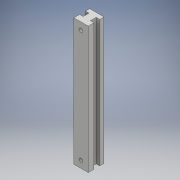
# Autodesk Inventor part: Screen Docking rail
Saved by Autodesk Inventor 2018 (Build 220112000, 112)
## iProperties
Created: 2018-05-10
Part Number: Screen Docking rail
Material: Generic
Document SubType Name: Modeling
Designer: Jasper
Density: 1 g/cm^3
Appearance: Default
Author: Jasper
Autodesk Inventor part; units mm, degrees
ref_plane "YZ Plane" through (0, 0, 0) normal (1, 0, 0) x (0, 1, 0)
ref_plane "XZ Plane" through (0, 0, 0) normal (0, 1, 0) x (-1, 0, 0)
ref_plane "XY Plane" through (0, 0, 0) normal (0, 0, 1) x (1, 0, 0)
sketch "Sketch1" plane through (0, 0, 0) normal (0, 1, 0) x (-1, 0, 0)
  line L0 (-5, 44.25) -> (5, 44.25)
  line L1 (5, 44.25) -> (5, -44.25)
  line L2 (5, -44.25) -> (-5, -44.25)
  line L3 (-5, -44.25) -> (-5, 44.25)
  line L4 (-5, 44.25) -> (5, -44.25) construction
  line L5 (5, 44.25) -> (-5, -44.25) construction
  point P0 (0, 0)
  dimension "d0" = 88.5
  dimension "d1" = 10
  constraints: 12 end point, 2 midpoint, 2 parallel, 1 horizontal, 1 perpendicular
  measures "d0" distance of L0.end L1.end
  measures "d1" distance of L1.end L2.end
extrude "Extrusion1" add sketch "Sketch1" along normal blind 11
sketch "Sketch2" plane through (-5, 0, 44.25) normal (0, 0, 1) x (1, 0, 0)
  line L0 (10, 0) -> (0, 0) projected
  line L1 (5, 0) -> (0, 0)
  line L2 (0, 0) -> (0, 4)
  line L3 (0, 4) -> (2.5, 4)
  line L4 (2.5, 4) -> (2.5, 8)
  line L5 (2.5, 8) -> (0, 8)
  line L6 (0, 8) -> (0, 11)
  line L7 (0, 11) -> (5, 11)
  line L8 (0, 11) -> (10, 11) projected
  line L9 (5, 11) -> (5, 0) construction
  line L10 (0, 0) -> (10, 0)
  line L11 (10, 0) -> (10, 4)
  line L12 (10, 4) -> (7.5, 4)
  line L13 (7.5, 4) -> (7.5, 8)
  line L14 (7.5, 8) -> (10, 8)
  line L15 (10, 8) -> (10, 11)
  line L16 (10, 11) -> (5, 11)
  dimension "d4" = 3
  dimension "d5" = 4
  dimension "d6" = 2.5
  constraints: 30 end point, 7 symmetric about line, 4 perpendicular, 4 point on line, 2 horizontal, 2 midpoint, 1 vertical
  measures "d4" distance of L6.end L5.end
  measures "d5" distance of L0.end L2.end
  measures "d6" distance of L2.end L3.end
extrude "Extrusion2" cut sketch "Sketch2" against normal through all keep common part
sketch "Sketch3" plane through (0, 0, 0) normal (0, -1, 0) x (1, 0, 0)
  line L0 (0, 0) -> (0, 39.25) construction
  circle A0 centre (0, 39.25) radius 1.25
  line L1 (5, -44.25) -> (5, 44.25) construction
  line L2 (5, 0) -> (-5, 0) construction
  line L3 (-5, 44.25) -> (-5, -44.25) construction
  circle A1 centre (0, -39.25) radius 1.25
  dimension "d9" = 2.5
  dimension "d10" = 39.25
  constraints: 4 end point, 2 centre point, 2 midpoint, 1 coincident, 1 symmetric about line, 1 vertical, 1 other
  measures "d9" diameter of A0
  measures "d10" distance of L0.start L0.end
extrude "Extrusion3" cut sketch "Sketch3" against normal blind 4
sketch "Sketch4" plane through (0, 11, 0) normal (0, 1, 0) x (1, 0, 0)
  line L0 (-2, 11) -> (2, 11)
  line L1 (2, 11) -> (2, -9)
  line L2 (2, -9) -> (-2, -9)
  line L3 (-2, -9) -> (-2, 11)
  line L4 (-2, 11) -> (2, -9) construction
  line L5 (2, 11) -> (-2, -9) construction
  line L6 (0, 1) -> (0, 0) construction
  dimension "d13" = 4
  dimension "d14" = 20
  dimension "d15" = 1
  constraints: 14 end point, 2 midpoint, 2 parallel, 1 horizontal, 1 perpendicular, 1 vertical
  measures "d13" distance of L0.start L0.end
  measures "d14" distance of L2.end L0.start
  measures "d15" distance of L6.start L6.end
extrude "Extrusion4" cut sketch "Sketch4" against normal blind 4.7
sketch "Sketch5" plane through (0, 11, 0) normal (0, 1, 0) x (1, 0, 0)
  line L0 (-2, -9) -> (-2, 11) projected
  line L1 (-2, 11) -> (2, 11) projected
  line L2 (2, 11) -> (2, -9) projected
  line L3 (-1.5, -9) -> (-1.5, 10.5)
  line L4 (-1.5, 10.5) -> (1.5, 10.5)
  line L5 (1.5, 10.5) -> (1.5, -9)
  line L6 (-1.5, -9) -> (1.5, -9)
  line L7 (2, -9) -> (-2, -9) projected
  point P0 (0, 0)
  dimension "d18" = 0.5
  constraints: 8 end point, 1 collinear, 1 horizontal, 2 other
  measures "d18" distance between parallel lines of L0 L3
extrude "Extrusion5" add sketch "Sketch5" against normal blind 0.6 contours L3 L4 L5 L6
fillet "Fillet1" radius 4 1 edges at (0, 10.4, 9)
sketch "Sketch7" plane through (0, 11, 0) normal (0, 1, 0) x (1, 0, 0)
  line L0 (1.5, 10.5) -> (-1.5, 10.5) construction
  line L1 (-1.5, 10.5) -> (1.5, 10.5) construction
  line L2 (1.5, 10.5) -> (1.5, 7.5) construction
  line L3 (1.5, 7.5) -> (-1.5, 7.5) construction
  line L4 (-1.5, 7.5) -> (-1.5, 10.5) construction
  line L5 (1.5, -9) -> (1.5, 10.5) projected
  line L6 (-1.5, 10.5) -> (1.5, 7.5) construction
  circle A0 centre (0, 9) radius 1.5
  line L7 (0, 9) -> (1.5, 9)
  line L8 (0, 9) -> (-1.5, 9)
  point P0 (0, 0)
  dimension "d24" = 3
  dimension "d25" = 3
  constraints: 14 end point, 2 midpoint, 2 parallel, 2 point on circle, 1 centre point, 1 collinear, 1 horizontal, 1 perpendicular, 1 point on line
  measures "d24" distance of L1.end L2.end
  measures "d25" diameter of A0
revolve "Revolution1" add sketch "Sketch7" angle 180 about axis through (0, 11, -9) along (1, 0, 0) picked at (0.9282, 9.352) contours L7 L8 A0
sketch "Sketch8" plane through (0, 6.3, 0) normal (0, 1, 0) x (1, 0, 0)
  line L0 (0, 10.5) -> (-1.5, 10.5) projected
  line L1 (1.5, 10.5) -> (0, 10.5) projected
  line L2 (1.5, 10.5) -> (-1.5, 10.5)
  line L3 (-1.5, 10.5) -> (-1.5, 10)
  line L4 (-1.5, 10) -> (1.5, 10)
  line L5 (1.5, 10) -> (1.5, 10.5)
  point P0 (0, 0)
  dimension "d27" = 0.5
  constraints: 8 end point, 2 parallel, 1 horizontal, 1 perpendicular
  measures "d27" distance of L2.end L3.end
extrude "Extrusion7" add sketch "Sketch8" along normal up to surface (4.1 mm away)
sketch "Sketch9" plane through (-1.5, 6.3, -10) normal (0, 0, 1) x (1, 0, 0)
  line L0 (0, 0) -> (0, 4.1) projected
  line L1 (0, 4.1) -> (3, 4.1)
  line L2 (3, 4.1) -> (3, 4)
  line L3 (3, 4) -> (0, 4)
  line L4 (0, 4) -> (0, 4.1)
  point P0 (1.5, -6.3)
  dimension "d30" = 0.1
  constraints: 8 end point, 2 parallel, 1 horizontal, 1 perpendicular
  measures "d30" distance of L1.end L2.end
extrude "Extrusion8" cut sketch "Sketch9" against normal up to next
sketch "Sketch10" plane through (0, 10.4, 0) normal (0, -1, 0) x (1, 0, 0)
  line L0 (1.5, -10.5) -> (1.5, 5) projected
  line L1 (-1.5, 5) -> (-1.5, -10.5) projected
  line L2 (1.5, -10.5) -> (-1.5, -10.5) projected
  line L3 (-2, 5) -> (-2, -11)
  line L4 (-2, -11) -> (2, -11)
  line L5 (2, -11) -> (2, 5)
  line L6 (2, 5) -> (1.5, 5)
  line L7 (5, 44.25) -> (5, -44.25) projected
  line L8 (-2, 5) -> (-1.5, 5)
  point P0 (0, 0)
  dimension "d33" = 0.5
  constraints: 10 end point, 1 collinear, 1 perpendicular, 2 other
  measures "d33" distance between parallel lines of L1 L3
extrude "Extrusion9" add sketch "Sketch10" against normal blind 0.2
body "Solid1"
